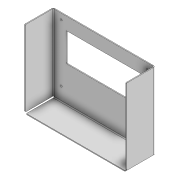
# Autodesk Inventor part: Display_Mount_B
Saved by Autodesk Inventor 2020 (Build 240168000, 168)
## iProperties
Created: 2021-12-05
Part Number: Display_Mount_B
Material: 一般
Document SubType Name: Sheet Metal
Designer: ken113
Density: 1 g/cm^3
Sheet Metal Rule: Default_mm
Appearance: 既定
Author: ken113
Autodesk Inventor part; units mm, degrees
ref_plane "YZ Plane" through (0, 0, 0) normal (1, 0, 0) x (0, 1, 0)
ref_plane "XZ Plane" through (0, 0, 0) normal (0, 1, 0) x (-1, 0, 0)
ref_plane "XY Plane" through (0, 0, 0) normal (0, 0, 1) x (1, 0, 0)
sketch "スケッチ1" plane through (0, 0, 0) normal (0, 0, 1) x (1, 0, 0)
  line L0 (172, -132) -> (-172, -132)
  line L1 (-172, -132) -> (-172, 132)
  line L2 (-172, 132) -> (172, 132)
  line L3 (172, 132) -> (172, -132)
  line L4 (172, -132) -> (-172, 132) construction
  line L5 (-172, -132) -> (172, 132) construction
  point P0 (0, 0)
  dimension "d0" = 264
  dimension "d1" = 344
  measures "d0" distance of L0.end L1.end
  measures "d1" distance of L1.end L2.end
extrude "プレート1" add sketch "スケッチ1" along normal blind 3
sketch "スケッチ2" plane through (172, -135, 6) normal (0, -1, 0) x (1, 0, 0)
  line L0 (-344, 0) -> (0, 0)
  line L1 (0, 0) -> (0, 94)
  line L2 (0, 94) -> (-344, 94)
  line L3 (-344, 94) -> (-344, 0)
  constraints: 6 end point, 1 horizontal, 1 perpendicular, 1 vertical
edge flange "フランジ1" height 100 angle 90 thickness 3 bend radius 3 thickness toward (0, -1, 0) relief straight relief width 3 relief depth 1.5 edges at (0, -132, 3) wall of the first edge with corners at (-172, -135, 6) (172, -135, 6) (172, -135, 100) (-172, -135, 100)
bend "曲げ1"
corner "コーナー1"
sketch "スケッチ3" plane through (0, 0, 3) normal (0, 0, 1) x (1, 0, 0)
  line L0 (153, -88) -> (-147, -88)
  line L1 (-147, -88) -> (-147, 112)
  line L2 (-147, 112) -> (153, 112)
  line L3 (153, 112) -> (153, -88)
  line L4 (153, -88) -> (-147, 112) construction
  line L5 (-147, -88) -> (153, 112) construction
  line L6 (172, -132) -> (-172, -132) projected
  line L7 (-172, 132) -> (172, 132) projected
  point P0 (0, 0)
  point P1 (3, 12)
  dimension "d13" = 300
  dimension "d14" = 200
  dimension "d51" = 120
  constraints: 12 end point, 2 midpoint, 2 parallel, 1 horizontal, 1 perpendicular
  measures "d13" distance of L0.start L0.end
  measures "d14" distance of L0.end L1.end
  measures "d51" distance from line of L7 point (3, 12)
hole "穴1" at (-147, 112, 3) at (-147, -88, 3) at (153, -88, 3) at (153, 112, 3) direction (0, 0, -1) diameter 6.2 depth 3 tip angle 118
sketch "スケッチ4" plane through (0, 0, 3) normal (0, 0, 1) x (1, 0, 0)
  line L0 (130, -11.8) -> (-130, -11.8)
  line L1 (-130, -11.8) -> (-130, 88.2)
  line L2 (-130, 88.2) -> (130, 88.2)
  line L3 (130, 88.2) -> (130, -11.8)
  line L4 (130, -11.8) -> (-130, 88.2) construction
  line L5 (-130, -11.8) -> (130, 88.2) construction
  circle A0 centre (-147, 112) radius 3.1 projected
  point P0 (0, 0)
  point P1 (0, 38.2)
  point P2 (0, 38.2)
  dimension "d23" = 100
  dimension "d24" = 23.8
  dimension "d25" = 260
  constraints: 12 end point, 3 midpoint, 2 parallel, 1 horizontal, 1 perpendicular, 1 vertical alignment
  measures "d23" distance of L2.end L0.start
  measures "d24" distance from line of L2 A0.centre
  measures "d25" distance of L1.end L2.end
extrude "押し出し1" cut sketch "スケッチ4" against normal through all contours L0 L1 L2 L3
fillet "フィレット1" radius 2 4 edges at (130, -11.8, 1.5) (130, 88.2, 1.5) (-130, 88.2, 1.5) (-130, -11.8, 1.5)
sketch "スケッチ6" plane through (175, 132, 6) normal (1, 0, 0) x (0, 1, 0)
  line L0 (-264, 0) -> (0, 0)
  line L1 (0, 0) -> (0, 94)
  line L2 (0, 94) -> (-264, 94)
  line L3 (-264, 94) -> (-264, 0)
  constraints: 6 end point, 1 horizontal, 1 perpendicular, 1 vertical
edge flange "フランジ2" height 100 angle 90 thickness 3 bend radius 3 thickness toward (1, 0, 0) relief straight relief width 3 relief depth 1.5 corner gap 3 corner form 0 edges at (172, 0, 3) (-172, 0, 3) wall of the first edge with corners at (175, -132, 6) (175, 132, 6) (175, 132, 100) (175, -132, 100)
bend "曲げ2"
corner "コーナー2"
fillet "フィレット2" radius 2 6 edges at (-176.5, 132, 100) (-176.5, -132, 100) (-172, -136.5, 100) (172, -136.5, 100) (176.5, -132, 100) (176.5, 132, 100)
equation "\"d21\" = Thickness"
equation "\"d2\" = Thickness"
equation "\"d3\" = BendReliefWidth"
equation "\"d4\" = BendReliefDepth"
equation "\"d5\" = MinimumRemnant"
equation "\"d6\" = TransitionRadius"
equation "\"d9\" = BendRadius"
equation "\"d10\" = CornerReliefSize"
equation "\"d11\" = GapSize"
equation "\"d12\" = JacobiRadiusSize"
equation "\"d40\" = BendReliefWidth"
equation "\"d41\" = BendReliefDepth"
equation "\"d42\" = MinimumRemnant"
equation "\"d43\" = TransitionRadius"
equation "\"d46\" = BendRadius"
equation "\"d47\" = CornerReliefSize"
equation "\"d48\" = GapSize"
equation "\"d49\" = JacobiRadiusSize"
equation "\"BendRadius\" = Thickness"
equation "\"BendReliefWidth\" = Thickness"
equation "\"BendReliefDepth\" = 0.5 * Thickness"
equation "\"CornerReliefSize\" = 4 * Thickness"
equation "\"MinimumRemnant\" = 2 * Thickness"
equation "\"TransitionRadius\" = BendRadius"
equation "\"JacobiRadiusSize\" = BendRadius"
equation "\"GapSize\" = Thickness"
equation "\"Thickness\" = 3"
